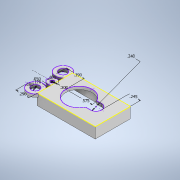
# Autodesk Inventor part: Back Half Torso
Saved by Autodesk Inventor 2020 (Build 240168000, 168)
## iProperties
Created: 2022-04-29
Part Number: Back Half Torso
Material: Generic
Document SubType Name: Modeling
Designer: Administrator
Density: 1 g/cm^3
Appearance: Default
Author: Administrator
Autodesk Inventor part; units mm, degrees
ref_plane "YZ Plane" through (0, 0, 0) normal (1, 0, 0) x (0, 1, 0)
ref_plane "XZ Plane" through (0, 0, 0) normal (0, 1, 0) x (-1, 0, 0)
ref_plane "XY Plane" through (0, 0, 0) normal (0, 0, 1) x (1, 0, 0)
sketch "Sketch1" plane through (0, 0, 0) normal (0, 0, 1) x (1, 0, 0)
  line L0 (0, 0) -> (-31.877, 0)
  line L1 (-31.877, 0) -> (-31.877, -5.969)
  line L2 (-31.877, -5.969) -> (0, -5.969)
  line L3 (0, -5.969) -> (0, 0)
  dimension "d0" = 31.877
  dimension "d1" = 5.969
  constraints: 8 end point, 2 parallel, 1 horizontal, 1 perpendicular
  measures "d0" distance of L2.end L1.end
  measures "d1" distance of L1.end L0.end
extrude "Extrusion1" add sketch "Sketch1" along normal blind 19.304
shell "Shell1" thickness 1.651 removed faces 1 at (-21.2513, -5.969, 12.8693)
sketch "Sketch2" plane through (-31.877, 0, 0) normal (0, 1, 0) x (1, 0, 0)
  arc A0 (19.8846, -6.604) -> (19.8846, -12.7) centre (13.2486, -9.652) ccw
  arc A1 (0, -7.5459) -> (0, -11.7581) centre (-1.4199, -9.652) ccw
  line L0 (0, 0) -> (0, -19.304) projected
  line L1 (0, 0) -> (0, -19.304) projected
  circle A2 centre (-1.4199, -9.652) radius 0.9525
  arc A3 (22.606, -12.7) -> (22.606, -6.604) centre (22.606, -9.652) ccw
  line L2 (31.877, 0) -> (31.877, -19.304) projected
  line L3 (22.606, -12.7) -> (19.8846, -12.7)
  line L4 (22.606, -6.604) -> (19.8846, -6.604)
  circle A4 centre (-3.175, -17.2678) radius 2.159
  arc A5 (0, -14.5321) -> (0.4881, -19.304) centre (-3.175, -17.2678) ccw
  line L5 (31.877, -19.304) -> (0, -19.304) construction
  line L6 (13.2486, -9.652) -> (-12.5267, -9.652) construction
  circle A6 centre (-3.175, -2.0362) radius 2.159
  arc A7 (0.4881, 0) -> (0, -4.7719) centre (-3.175, -2.0362) ccw
  line L7 (31.877, 0) -> (0, 0) projected
  line L8 (0, 0) -> (0, -19.304) projected
  line L9 (31.877, -19.304) -> (0, -19.304) projected
  line L10 (31.877, 0) -> (31.877, -19.304) projected
  point P0 (-3.9599, -9.652)
  point P1 (0, -9.652)
  point P2 (5.9461, -9.652)
  point P3 (13.2486, -2.3495)
  point P4 (25.654, -9.652)
  point P5 (-7.366, -17.2678)
  point P6 (-1.4199, -12.192)
  point P7 (-1.4199, -13.462)
  point P8 (0.4881, 0)
  point P9 (0, -4.7719)
  point P10 (0.4881, -19.304)
  point P11 (0, -14.5321)
  dimension "d5" = 14.605
  dimension "d6" = 5.08
  dimension "d8" = 1.905
  dimension "d11" = 9.906
  dimension "d12" = 6.223
  dimension "d13" = 6.096
  dimension "d16" = 4.318
  dimension "d17" = 2.032
  dimension "d18" = 7.366
  dimension "d19" = 1.27
  constraints: 17 point on circle, 8 centre point, 6 end point, 6 horizontal alignment, 4 point on line, 3 horizontal, 3 symmetric about line, 2 vertical alignment, 1 coincident, 1 midpoint, 1 tangent, 2 other
  measures "d5" diameter of A0
  measures "d6" diameter of A1
  measures "d8" diameter of A2
  measures "d11" distance of point (5.946, -9.652) point (-3.96, -9.652)
  measures "d12" distance from line of L2 point (25.654, -9.652)
  measures "d13" diameter of A3
  measures "d16" diameter of A4
  measures "d17" radial gap between concentric circles of A4 A5
  measures "d18" distance from line of L0 point (-7.366, -17.268)
  measures "d19" distance of point (-1.42, -13.462) point (-1.42, -12.192)
extrude "Extrusion2" add sketch "Sketch2" against normal blind 6.731 contours L0 A1
extrude "Extrusion3" cut sketch "Sketch2" against normal through all contours L4 A3 L3 A0
extrude "Extrusion4" add sketch "Sketch2" against normal blind 1.651 contours A7 L7 L0 | L0 L9 A5
body "Solid1"
